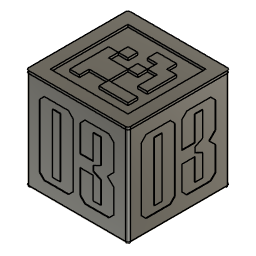
AutonOhm Apriltag 03 (Autodesk Fusion 360 design; units mm, degrees)
Autodesk Fusion 360 part; units mm, degrees
sketch "Skizze1" plane through (0, 0, 0) normal (0, 0, 1) x (1, 0, 0)
  line L0 (21, -21) -> (-21, -21)
  line L1 (-21, -21) -> (-21, 21)
  line L2 (-21, 21) -> (21, 21)
  line L3 (21, 21) -> (21, -21)
  line L4 (21, -21) -> (-21, 21) construction
  line L5 (-21, -21) -> (21, 21) construction
  dimension "d1" = 42
  dimension "d2" = 42
  constraint horizontal L0
  constraint perpendicular L0 L1
  constraint parallel L0 L2
  constraint parallel L1 L3
  constraint coincident L4 origin
  constraint coincident L5 origin
  measures "d1" distance of L1.end L2.end
  measures "d2" distance of L0.end L1.end
extrude "Extrusion1" add sketch "Skizze1" along normal blind 41 makes body 1
sketch "Skizze2" plane through (0, 0, 41) normal (0, 0, 1) x (-1, 0, 0)
  line L0 (-21, -21) -> (21, -21)
  line L1 (21, -21) -> (21, 21)
  line L2 (21, 21) -> (-21, 21)
  line L3 (-21, 21) -> (-21, -21)
  line L4 (21, -21) -> (-21, -21)
  line L5 (-21, -21) -> (-21, 21)
  line L6 (-21, 21) -> (21, 21)
  line L7 (21, 21) -> (21, -21)
  line L8 (-16, 16) -> (16, 16)
  line L9 (16, 16) -> (16, -16)
  line L10 (16, -16) -> (-16, -16)
  line L11 (-16, -16) -> (-16, 16)
  line L12 (-16, 16) -> (16, -16) construction
  line L13 (16, 16) -> (-16, -16) construction
  dimension "d5" = 32
  dimension "d6" = 32
  constraint horizontal L4
  constraint vertical L5
  constraint horizontal L6
  constraint vertical L7
  constraint coincident L2.end L3.start
  constraint coincident L0.end L1.start
  constraint horizontal L8
  constraint perpendicular L8 L9
  constraint parallel L8 L10
  constraint parallel L9 L11
  constraint coincident L12 origin
  constraint coincident L13 origin
  measures "d5" distance of L9.end L10.end
  measures "d6" distance of L8.end L9.end
extrude "Extrusion2" add sketch "Skizze2" along normal blind 1 separate body makes body 2
fillet "Abrundung1" radius 1 8 edges at (-21, 21, 20.5) (-21, -21, 20.5) (-21, 0, 0) (0, -21, 0) (21, -21, 20.5) (21, 0, 0) (21, 21, 20.5) (0, 21, 0) on bodies 1
fillet "Abrundung2" radius 1 1 edges at (21, 21, 41.5) on bodies 2
fillet "Abrundung3" radius 1 1 edges at (21, -21, 41.5) on bodies 2
fillet "Abrundung4" radius 1 1 edges at (-21, -21, 41.5) on bodies 2
fillet "Abrundung5" radius 1 1 edges at (-21, 21, 41.5) on bodies 2
sketch "Skizze3" plane through (0, 0, 0) normal (0, 0, -1) x (1, 0, 0)
  line L0 (-20, -20) -> (20, -20)
  line L1 (20, -20) -> (20, 20)
  line L2 (20, 20) -> (-20, 20)
  line L3 (-20, 20) -> (-20, -20)
  line L4 (-15.5554, -7.5319) -> (-15.5554, -12.9394)
  line L5 (-15.5554, -12.9394) -> (-1.7653, -13.0619)
  line L6 (-1.7653, -13.0619) -> (-1.8353, -7.8468)
  spline S0 degree 3 poles (-1.8353, -7.8468) (-9.4573, -5.9337) (-9.4543, 8.1703) (-0.2245, 8.2733) knots 0 0 0 0 1 1 1 1
  spline S1 degree 3 poles (-0.2245, 8.2733) (9.1628, 8.378) (10.5465, -5.8261) (1.9583, -7.8813) knots 0 0 0 0 1 1 1 1
  line L7 (1.9583, -7.8813) -> (1.9723, -13.0334)
  spline S2 degree 3 poles (1.9723, -13.0334) (15.5516, -12.9722) (18.9797, 12.8679) (-0.1523, 13.061) knots 0 0 0 0 1 1 1 1
  spline S3 degree 3 poles (-0.1523, 13.061) (-11.1806, 13.1724) (-15.9327, 2.2058) (-10.2013, -7.6521) knots 0 0 0 0 1 1 1 1
  line L8 (-10.2013, -7.6521) -> (-15.5554, -7.5319)
extrude "Extrusion3" add sketch "Skizze3" against normal blind 0.6 separate body contours L4 L5 L6 S0 S1 L7 S2 S3 L8 makes body 3
sketch "Skizze4" plane through (0, 0, 41) normal (0, 0, 1) x (-1, 0, 0)
  arc A0 (21, 20) -> (20, 21) centre (20, 20) ccw
  line L0 (20, 21) -> (-20, 21)
  arc A1 (-20, 21) -> (-21, 20) centre (-20, 20) ccw
  line L1 (-21, 20) -> (-21, -20)
  arc A2 (-21, -20) -> (-20, -21) centre (-20, -20) ccw
  line L2 (-20, -21) -> (20, -21)
  arc A3 (20, -21) -> (21, -20) centre (20, -20) ccw
  line L3 (21, -20) -> (21, 20)
  line L4 (21, 21) -> (-21, 21)
  line L5 (-21, 21) -> (-21, -21)
  line L6 (-21, -21) -> (21, -21)
  line L7 (21, -21) -> (21, 21)
  line L8 (20.0001, 19.9999) -> (-19.9999, 19.9999)
  line L9 (-19.9999, 19.9999) -> (-19.9999, -20.0001)
  line L10 (-19.9999, -20.0001) -> (20.0001, -20.0001)
  line L11 (20.0001, -20.0001) -> (20.0001, 19.9999)
  line L12 (-11.9999, 11.9999) -> (-11.9999, 8)
  line L13 (-11.9999, 8) -> (0, 8)
  line L14 (0, 8) -> (0, 0)
  line L15 (0, 0) -> (-4, 0)
  line L16 (-4, 0) -> (-4, -3.9999)
  line L17 (-4, -3.9999) -> (-8, -3.9999)
  line L18 (-8, -3.9999) -> (-8, 4)
  line L19 (-8, 4) -> (-11.9999, 4)
  line L20 (-11.9999, 4) -> (-11.9999, -7.9999)
  line L21 (-11.9999, -7.9999) -> (-8, -7.9999)
  line L22 (-8, -7.9999) -> (-8, -11.9999)
  line L23 (-8, -11.9999) -> (0, -11.9999)
  line L24 (0, -11.9999) -> (0, -7.9999)
  line L25 (0, -7.9999) -> (-4, -7.9999)
  line L26 (-4, -7.9999) -> (-4, -3.9999)
  line L27 (-4, -3.9999) -> (0, -3.9999)
  line L28 (0, -3.9999) -> (0, 0)
  line L29 (0, 0) -> (7.9999, 0)
  line L30 (7.9999, 0) -> (7.9999, -3.9999)
  line L31 (7.9999, -3.9999) -> (3.9999, -3.9999)
  line L32 (3.9999, -3.9999) -> (3.9999, -7.9999)
  line L33 (3.9999, -7.9999) -> (7.9999, -7.9999)
  line L34 (7.9999, -7.9999) -> (7.9999, -3.9999)
  line L35 (7.9999, -3.9999) -> (11.9999, -3.9999)
  line L36 (11.9999, -3.9999) -> (11.9999, 11.9999)
  line L37 (11.9999, 11.9999) -> (7.9999, 11.9999)
  line L38 (7.9999, 11.9999) -> (7.9999, 8)
  line L39 (7.9999, 8) -> (0, 8)
  line L40 (0, 8) -> (0, 11.9999)
  line L41 (0, 11.9999) -> (-11.9999, 11.9999)
extrude "Extrusion4" add sketch "Skizze4" along normal blind 1 separate body contours L12 L13 L40 L41 | L31 L32 L33 L34 | L17 L18 L19 L20 L21 L22 L23 L24 L25 L26 | L15 L16 L27 L28 | L14 L29 L30 L35 L36 L37 L38 L39 makes body 4 at (10.6666, 2.6666, 41)
sketch "Skizze5" plane through (0, -21, 0) normal (0, -1, 0) x (1, 0, 0)
  line L0 (-20, 41) -> (-20, 1)
  line L1 (-20, 1) -> (20, 1)
  line L2 (20, 1) -> (20, 41)
  line L3 (20, 41) -> (-20, 41)
  line L4 (21, 42) -> (-21, 42)
  line L5 (-21, 42) -> (-21, 0)
  line L6 (-21, 0) -> (21, 0)
  line L7 (21, 0) -> (21, 42)
  line L8 (20.0001, 40.9999) -> (-19.9999, 40.9999)
  line L9 (-19.9999, 40.9999) -> (-19.9999, 0.9999)
  line L10 (-19.9999, 0.9999) -> (20.0001, 0.9999)
  line L11 (20.0001, 0.9999) -> (20.0001, 40.9999)
  line L12 (21, 0) -> (21, 6)
  line L13 (21, 6) -> (-21, 6)
  line L14 (-21, 6) -> (-21, 0)
  line L15 (-21, 0) -> (21, 0)
  line L16 (-21, 42) -> (-21, 36)
  line L17 (-21, 36) -> (21, 36)
  line L18 (21, 36) -> (21, 42)
  line L19 (21, 42) -> (-21, 42)
  line L20 (-1.5965, 33.9045) -> (-3.5481, 35.9625)
  line L21 (-3.5481, 35.9625) -> (-13.5533, 35.9625)
  line L22 (-13.5533, 35.9625) -> (-15.5046, 33.9045)
  line L23 (-15.5046, 33.9045) -> (-15.5046, 7.9336)
  line L24 (-15.5046, 7.9336) -> (-13.5533, 5.9823)
  line L25 (-13.5533, 5.9823) -> (-3.5481, 5.9823)
  line L26 (-3.5481, 5.9823) -> (-1.5965, 7.9336)
  line L27 (-1.5965, 7.9336) -> (-1.5965, 33.9045)
  line L28 (-10.1473, 8.8205) -> (-10.1473, 33.124)
  line L29 (-10.1473, 33.124) -> (-6.9541, 33.124)
  line L30 (-6.9541, 33.124) -> (-6.9541, 8.8205)
  line L31 (-6.9541, 8.8205) -> (-10.1473, 8.8205)
  line L32 (15.1498, 17.9742) -> (12.4888, 20.5288)
  line L33 (12.4888, 20.5288) -> (15.1498, 23.1897)
  line L34 (15.1498, 23.1897) -> (15.1498, 33.9045)
  line L35 (15.1498, 33.9045) -> (13.0921, 35.9625)
  line L36 (13.0921, 35.9625) -> (3.2641, 35.9625)
  line L37 (3.2641, 35.9625) -> (1.2417, 33.9045)
  line L38 (1.2417, 33.9045) -> (1.2417, 22.9061)
  line L39 (1.2417, 22.9061) -> (6.5992, 22.9061)
  line L40 (6.5992, 22.9061) -> (6.5992, 33.124)
  line L41 (6.5992, 33.124) -> (9.7925, 33.124)
  line L42 (9.7925, 33.124) -> (9.7925, 22.977)
  line L43 (9.7925, 22.977) -> (6.6347, 21.4514)
  line L44 (6.6347, 21.4514) -> (6.6347, 19.3226)
  line L45 (6.6347, 19.3226) -> (9.7925, 17.797)
  line L46 (9.7925, 17.797) -> (9.7925, 8.8205)
  line L47 (9.7925, 8.8205) -> (6.5992, 8.8205)
  line L48 (6.5992, 8.8205) -> (6.5992, 17.9742)
  line L49 (6.5992, 17.9742) -> (1.2417, 17.9742)
  line L50 (1.2417, 17.9742) -> (1.2417, 8.0399)
  line L51 (1.2417, 8.0399) -> (3.2641, 5.9823)
  line L52 (3.2641, 5.9823) -> (13.0921, 5.9823)
  line L53 (13.0921, 5.9823) -> (15.1498, 8.0399)
  line L54 (15.1498, 8.0399) -> (15.1498, 17.9742)
extrude "Extrusion5" cut sketch "Skizze5" against normal blind 0.2 contours L13 L20 L21 L22 L23 L24 L26 L27 | L13 L32 L33 L34 L35 L36 L37 L38 L39 L40 L41 L42 L43 L44 L45 L46 L47 L48 L49 L50 L51 L53 L54 bodies 1
sketch "Skizze6" plane through (-21, 0, 0) normal (-1, 0, 0) x (0, -1, 0)
  line L0 (20, 1) -> (20, 41)
  line L1 (20, 41) -> (-20, 41)
  line L2 (-20, 41) -> (-20, 1)
  line L3 (-20, 1) -> (20, 1)
  line L4 (21, 42) -> (-21, 42)
  line L5 (-21, 42) -> (-21, 0)
  line L6 (-21, 0) -> (21, 0)
  line L7 (21, 0) -> (21, 42)
  line L8 (20.0001, 40.9999) -> (-19.9999, 40.9999)
  line L9 (-19.9999, 40.9999) -> (-19.9999, 0.9999)
  line L10 (-19.9999, 0.9999) -> (20.0001, 0.9999)
  line L11 (20.0001, 0.9999) -> (20.0001, 40.9999)
  line L12 (21, 0) -> (21, 6)
  line L13 (21, 6) -> (-21, 6)
  line L14 (-21, 6) -> (-21, 0)
  line L15 (-21, 0) -> (21, 0)
  line L16 (-21, 42) -> (-21, 36)
  line L17 (-21, 36) -> (21, 36)
  line L18 (21, 36) -> (21, 42)
  line L19 (21, 42) -> (-21, 42)
  line L20 (-1.5965, 33.9045) -> (-3.5481, 35.9625)
  line L21 (-3.5481, 35.9625) -> (-13.5533, 35.9625)
  line L22 (-13.5533, 35.9625) -> (-15.5046, 33.9045)
  line L23 (-15.5046, 33.9045) -> (-15.5046, 7.9336)
  line L24 (-15.5046, 7.9336) -> (-13.5533, 5.9823)
  line L25 (-13.5533, 5.9823) -> (-3.5481, 5.9823)
  line L26 (-3.5481, 5.9823) -> (-1.5965, 7.9336)
  line L27 (-1.5965, 7.9336) -> (-1.5965, 33.9045)
  line L28 (-10.1473, 8.8205) -> (-10.1473, 33.124)
  line L29 (-10.1473, 33.124) -> (-6.9541, 33.124)
  line L30 (-6.9541, 33.124) -> (-6.9541, 8.8205)
  line L31 (-6.9541, 8.8205) -> (-10.1473, 8.8205)
  line L32 (15.1498, 17.9742) -> (12.4888, 20.5288)
  line L33 (12.4888, 20.5288) -> (15.1498, 23.1897)
  line L34 (15.1498, 23.1897) -> (15.1498, 33.9045)
  line L35 (15.1498, 33.9045) -> (13.0921, 35.9625)
  line L36 (13.0921, 35.9625) -> (3.2641, 35.9625)
  line L37 (3.2641, 35.9625) -> (1.2417, 33.9045)
  line L38 (1.2417, 33.9045) -> (1.2417, 22.9061)
  line L39 (1.2417, 22.9061) -> (6.5992, 22.9061)
  line L40 (6.5992, 22.9061) -> (6.5992, 33.124)
  line L41 (6.5992, 33.124) -> (9.7925, 33.124)
  line L42 (9.7925, 33.124) -> (9.7925, 22.977)
  line L43 (9.7925, 22.977) -> (6.6347, 21.4514)
  line L44 (6.6347, 21.4514) -> (6.6347, 19.3226)
  line L45 (6.6347, 19.3226) -> (9.7925, 17.797)
  line L46 (9.7925, 17.797) -> (9.7925, 8.8205)
  line L47 (9.7925, 8.8205) -> (6.5992, 8.8205)
  line L48 (6.5992, 8.8205) -> (6.5992, 17.9742)
  line L49 (6.5992, 17.9742) -> (1.2417, 17.9742)
  line L50 (1.2417, 17.9742) -> (1.2417, 8.0399)
  line L51 (1.2417, 8.0399) -> (3.2641, 5.9823)
  line L52 (3.2641, 5.9823) -> (13.0921, 5.9823)
  line L53 (13.0921, 5.9823) -> (15.1498, 8.0399)
  line L54 (15.1498, 8.0399) -> (15.1498, 17.9742)
extrude "Extrusion6" cut sketch "Skizze6" against normal blind 0.2 contours L13 L32 L33 L34 L35 L36 L37 L38 L39 L40 L41 L42 L43 L44 L45 L46 L47 L48 L49 L50 L51 L53 L54 | L13 L20 L21 L22 L23 L24 L26 L27 bodies 1
sketch "Skizze7" plane through (0, 21, 0) normal (0, 1, 0) x (-1, 0, 0)
  line L0 (20, 1) -> (20, 41)
  line L1 (20, 41) -> (-20, 41)
  line L2 (-20, 41) -> (-20, 1)
  line L3 (-20, 1) -> (20, 1)
  line L4 (21, 42) -> (-21, 42)
  line L5 (-21, 42) -> (-21, 0)
  line L6 (-21, 0) -> (21, 0)
  line L7 (21, 0) -> (21, 42)
  line L8 (20.0001, 40.9999) -> (-19.9999, 40.9999)
  line L9 (-19.9999, 40.9999) -> (-19.9999, 0.9999)
  line L10 (-19.9999, 0.9999) -> (20.0001, 0.9999)
  line L11 (20.0001, 0.9999) -> (20.0001, 40.9999)
  line L12 (21, 0) -> (21, 6)
  line L13 (21, 6) -> (-21, 6)
  line L14 (-21, 6) -> (-21, 0)
  line L15 (-21, 0) -> (21, 0)
  line L16 (-21, 42) -> (-21, 36)
  line L17 (-21, 36) -> (21, 36)
  line L18 (21, 36) -> (21, 42)
  line L19 (21, 42) -> (-21, 42)
  line L20 (-1.5965, 33.9045) -> (-3.5481, 35.9625)
  line L21 (-3.5481, 35.9625) -> (-13.5533, 35.9625)
  line L22 (-13.5533, 35.9625) -> (-15.5046, 33.9045)
  line L23 (-15.5046, 33.9045) -> (-15.5046, 7.9336)
  line L24 (-15.5046, 7.9336) -> (-13.5533, 5.9823)
  line L25 (-13.5533, 5.9823) -> (-3.5481, 5.9823)
  line L26 (-3.5481, 5.9823) -> (-1.5965, 7.9336)
  line L27 (-1.5965, 7.9336) -> (-1.5965, 33.9045)
  line L28 (-10.1473, 8.8205) -> (-10.1473, 33.124)
  line L29 (-10.1473, 33.124) -> (-6.9541, 33.124)
  line L30 (-6.9541, 33.124) -> (-6.9541, 8.8205)
  line L31 (-6.9541, 8.8205) -> (-10.1473, 8.8205)
  line L32 (15.1498, 17.9742) -> (12.4888, 20.5288)
  line L33 (12.4888, 20.5288) -> (15.1498, 23.1897)
  line L34 (15.1498, 23.1897) -> (15.1498, 33.9045)
  line L35 (15.1498, 33.9045) -> (13.0921, 35.9625)
  line L36 (13.0921, 35.9625) -> (3.2641, 35.9625)
  line L37 (3.2641, 35.9625) -> (1.2417, 33.9045)
  line L38 (1.2417, 33.9045) -> (1.2417, 22.9061)
  line L39 (1.2417, 22.9061) -> (6.5992, 22.9061)
  line L40 (6.5992, 22.9061) -> (6.5992, 33.124)
  line L41 (6.5992, 33.124) -> (9.7925, 33.124)
  line L42 (9.7925, 33.124) -> (9.7925, 22.977)
  line L43 (9.7925, 22.977) -> (6.6347, 21.4514)
  line L44 (6.6347, 21.4514) -> (6.6347, 19.3226)
  line L45 (6.6347, 19.3226) -> (9.7925, 17.797)
  line L46 (9.7925, 17.797) -> (9.7925, 8.8205)
  line L47 (9.7925, 8.8205) -> (6.5992, 8.8205)
  line L48 (6.5992, 8.8205) -> (6.5992, 17.9742)
  line L49 (6.5992, 17.9742) -> (1.2417, 17.9742)
  line L50 (1.2417, 17.9742) -> (1.2417, 8.0399)
  line L51 (1.2417, 8.0399) -> (3.2641, 5.9823)
  line L52 (3.2641, 5.9823) -> (13.0921, 5.9823)
  line L53 (13.0921, 5.9823) -> (15.1498, 8.0399)
  line L54 (15.1498, 8.0399) -> (15.1498, 17.9742)
extrude "Extrusion7" cut sketch "Skizze7" against normal blind 0.2 contours L13 L32 L33 L34 L35 L36 L37 L38 L39 L40 L41 L42 L43 L44 L45 L46 L47 L48 L49 L50 L51 L53 L54 | L13 L20 L21 L22 L23 L24 L26 L27 bodies 1
sketch "Skizze8" plane through (21, 0, 0) normal (1, 0, 0) x (0, 1, 0)
  line L0 (-20, 41) -> (-20, 1)
  line L1 (-20, 1) -> (20, 1)
  line L2 (20, 1) -> (20, 41)
  line L3 (20, 41) -> (-20, 41)
  line L4 (21, 42) -> (-21, 42)
  line L5 (-21, 42) -> (-21, 0)
  line L6 (-21, 0) -> (21, 0)
  line L7 (21, 0) -> (21, 42)
  line L8 (20.0001, 40.9999) -> (-19.9999, 40.9999)
  line L9 (-19.9999, 40.9999) -> (-19.9999, 0.9999)
  line L10 (-19.9999, 0.9999) -> (20.0001, 0.9999)
  line L11 (20.0001, 0.9999) -> (20.0001, 40.9999)
  line L12 (21, 0) -> (21, 6)
  line L13 (21, 6) -> (-21, 6)
  line L14 (-21, 6) -> (-21, 0)
  line L15 (-21, 0) -> (21, 0)
  line L16 (-21, 42) -> (-21, 36)
  line L17 (-21, 36) -> (21, 36)
  line L18 (21, 36) -> (21, 42)
  line L19 (21, 42) -> (-21, 42)
  line L20 (-1.5965, 33.9045) -> (-3.5481, 35.9625)
  line L21 (-3.5481, 35.9625) -> (-13.5533, 35.9625)
  line L22 (-13.5533, 35.9625) -> (-15.5046, 33.9045)
  line L23 (-15.5046, 33.9045) -> (-15.5046, 7.9336)
  line L24 (-15.5046, 7.9336) -> (-13.5533, 5.9823)
  line L25 (-13.5533, 5.9823) -> (-3.5481, 5.9823)
  line L26 (-3.5481, 5.9823) -> (-1.5965, 7.9336)
  line L27 (-1.5965, 7.9336) -> (-1.5965, 33.9045)
  line L28 (-10.1473, 8.8205) -> (-10.1473, 33.124)
  line L29 (-10.1473, 33.124) -> (-6.9541, 33.124)
  line L30 (-6.9541, 33.124) -> (-6.9541, 8.8205)
  line L31 (-6.9541, 8.8205) -> (-10.1473, 8.8205)
  line L32 (15.1498, 17.9742) -> (12.4888, 20.5288)
  line L33 (12.4888, 20.5288) -> (15.1498, 23.1897)
  line L34 (15.1498, 23.1897) -> (15.1498, 33.9045)
  line L35 (15.1498, 33.9045) -> (13.0921, 35.9625)
  line L36 (13.0921, 35.9625) -> (3.2641, 35.9625)
  line L37 (3.2641, 35.9625) -> (1.2417, 33.9045)
  line L38 (1.2417, 33.9045) -> (1.2417, 22.9061)
  line L39 (1.2417, 22.9061) -> (6.5992, 22.9061)
  line L40 (6.5992, 22.9061) -> (6.5992, 33.124)
  line L41 (6.5992, 33.124) -> (9.7925, 33.124)
  line L42 (9.7925, 33.124) -> (9.7925, 22.977)
  line L43 (9.7925, 22.977) -> (6.6347, 21.4514)
  line L44 (6.6347, 21.4514) -> (6.6347, 19.3226)
  line L45 (6.6347, 19.3226) -> (9.7925, 17.797)
  line L46 (9.7925, 17.797) -> (9.7925, 8.8205)
  line L47 (9.7925, 8.8205) -> (6.5992, 8.8205)
  line L48 (6.5992, 8.8205) -> (6.5992, 17.9742)
  line L49 (6.5992, 17.9742) -> (1.2417, 17.9742)
  line L50 (1.2417, 17.9742) -> (1.2417, 8.0399)
  line L51 (1.2417, 8.0399) -> (3.2641, 5.9823)
  line L52 (3.2641, 5.9823) -> (13.0921, 5.9823)
  line L53 (13.0921, 5.9823) -> (15.1498, 8.0399)
  line L54 (15.1498, 8.0399) -> (15.1498, 17.9742)
extrude "Extrusion8" cut sketch "Skizze8" against normal blind 0.2 contours L13 L20 L21 L22 L23 L24 L26 L27 | L13 L32 L33 L34 L35 L36 L37 L38 L39 L40 L41 L42 L43 L44 L45 L46 L47 L48 L49 L50 L51 L53 L54 bodies 1
named bodies: "Grundkörper", "Apriltag Kranz", "OhmLogo Unterseite"
